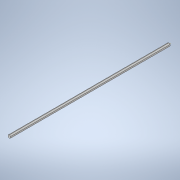
# Autodesk Inventor part: 5mm axel
Saved by Autodesk Inventor 2021 (Build 250183000, 183)
## iProperties
Created: 2016-09-04
Part Number: 5mm axel
Material: Generic
Description: STEP AP203
Document SubType Name: Modeling
Designer: User
Density: 1 g/cm^3
Appearance: Default
Mass: 1.34049 g
Surface Area: 11.1245 cm^2
Volume: 1.34049 cm^3
Sending System: SolidWorks 2015
Preprocessor: SwSTEP 2.0
Title: REV-41-1349_Default.step
Revision Number: ANY
Autodesk Inventor part; units mm, degrees
ref_plane "YZ Plane" through (0, 0, 0) normal (1, 0, 0) x (0, 1, 0)
ref_plane "XZ Plane" through (0, 0, 0) normal (0, 1, 0) x (-1, 0, 0)
ref_plane "XY Plane" through (0, 0, 0) normal (0, 0, 1) x (1, 0, 0)
sketch "Sketch1" plane through (-2.1, -1.2124, 67.5) normal (0, 0, 1) x (1, 0, 0)
  line L0 (2.1, 4.0992) -> (4.6, 2.6558) projected
  line L1 (2.1, 3.6373) -> (0, 2.4249) projected
  line L2 (-0.4, 2.6558) -> (2.1, 4.0992) projected
  line L3 (-0.4, -0.2309) -> (-0.4, 2.6558) projected
  line L4 (2.1, -1.6743) -> (-0.4, -0.2309) projected
  line L5 (4.6, -0.2309) -> (2.1, -1.6743) projected
  line L6 (4.6, 2.6558) -> (4.6, -0.2309) projected
  point P0 (2.1, 1.2124)
extrude "Extrusion1" add sketch "Sketch1" against normal blind 317.5
sketch "Sketch2" plane through (-2.1, -1.2124, -250) normal (0, 0, -1) x (1, 0, 0)
  point P0 (2.1, -1.2124)
  point P1 (2.1, -1.2124)
  constraints: 1 coincident
body "Solid2"
